Autodesk Fusion 360 part; units mm, degrees
note: some values were not read from the file. Chosen so that the rebuilt part matches the saved one: a side.
(part 2 of 2)
  spline S329 degree 2 poles (-148.7917, 5.9755) (-148.7208, 5.8468) (-148.7208, 5.7496) knots 0 0 0 1 1 1
  spline S330 degree 2 poles (-152.9965, 5.5659) (-152.9965, 5.6841) (-152.944, 5.9416) knots 0 0 0 1 1 1
  spline S331 degree 2 poles (-152.2034, 5.2611) (-151.8751, 5.2611) (-151.3288, 5.8134) knots 0 0 0 1 1 1
  spline S332 degree 2 poles (-160.0589, 6.9971) (-159.4128, 6.3957) (-159.4128, 5.9177) knots 0 0 0 1 1 1
  spline S333 degree 2 poles (-153.6965, 5.7036) (-153.3774, 6.0595) (-152.6498, 7.2204) knots 0 0 0 1 1 1
  spline S334 degree 2 poles (-164.6656, 7.3964) (-164.4713, 7.5592) (-164.2664, 7.5592) knots 0 0 0 1 1 1
  spline S335 degree 2 poles (-153.5323, 5.4568) (-154.0812, 4.8698) (-154.5041, 4.8698) knots 0 0 0 1 1 1
  spline S336 degree 2 poles (-158.3307, 4.1265) (-158.3964, 3.7982) (-158.3964, 3.5539) knots 0 0 0 1 1 1
  spline S337 degree 2 poles (-160.0563, 8.6465) (-160.3767, 8.6465) (-160.596, 8.4482) knots 0 0 0 1 1 1
  spline S338 degree 2 poles (-163.2684, 5.395) (-162.3806, 6.8002) (-162.3071, 7.8507) knots 0 0 0 1 1 1
  line L109 (-160.2953, 7.2151) -> (-160.0589, 6.9971)
  spline S339 degree 2 poles (-162.3071, 7.8507) (-161.8475, 7.7824) (-161.8475, 7.5434) knots 0 0 0 1 1 1
  spline S340 degree 2 poles (-158.7326, 3.1862) (-158.9506, 3.1862) (-158.9506, 3.4331) knots 0 0 0 1 1 1
  spline S341 degree 2 poles (-163.1528, 5.0667) (-163.7043, 4.313) (-164.248, 3.8783) knots 0 0 0 1 1 1
  line L110 (-152.944, 5.9416) -> (-152.8862, 6.2306)
  spline S342 degree 2 poles (-154.659, 9.3399) (-154.2625, 9.3399) (-153.9657, 9.5369) knots 0 0 0 1 1 1
  spline S343 degree 2 poles (-152.403, 6.0666) (-152.4791, 5.6967) (-152.4791, 5.5864) knots 0 0 0 1 1 1
  spline S344 degree 2 poles (-154.6564, 5.7916) (-154.6564, 5.3478) (-154.3307, 5.3478) knots 0 0 0 1 1 1
  spline S345 degree 2 poles (-158.0576, 5.5053) (-157.7923, 5.1954) (-157.4063, 5.1954) knots 0 0 0 1 1 1
  spline S346 degree 2 poles (-157.4063, 5.1954) (-156.944, 5.1954) (-156.6196, 5.5841) knots 0 0 0 1 1 1
  spline S347 degree 2 poles (-156.9571, 7.4305) (-157.3248, 7.4305) (-157.7556, 7.0155) knots 0 0 0 1 1 1
  spline S348 degree 2 poles (-154.5041, 4.8698) (-154.8114, 4.8698) (-155.0005, 5.1074) knots 0 0 0 1 1 1
  spline S349 degree 2 poles (-152.4791, 5.5864) (-152.4791, 5.2611) (-152.2034, 5.2611) knots 0 0 0 1 1 1
  line L111 (-153.9657, 9.5369) -> (-154.575, 6.3773)
  spline S350 degree 2 poles (-156.2953, 6.5296) (-156.2953, 6.9315) (-156.4791, 7.181) knots 0 0 0 1 1 1
  spline S351 degree 2 poles (-154.5881, 8.9696) (-154.6906, 8.9538) (-154.7667, 8.9538) knots 0 0 0 1 1 1
  spline S352 degree 2 poles (-150.4607, 5.1508) (-150.659, 5.4318) (-150.659, 5.8757) knots 0 0 0 1 1 1
  line L112 (-155.1108, 6.3379) -> (-154.5881, 8.9696)
  spline S353 degree 2 poles (-155.0005, 5.1074) (-155.1896, 5.3451) (-155.1896, 5.7286) knots 0 0 0 1 1 1
sketch "Sketch4" plane through (-20, 0, 0) normal (-1, 0, 0) x (0, -1, 0)
  spline S0 degree 2 poles (168.3547, 5.852) (168.3547, 5.4239) (168.5898, 5.1797) knots 0 0 0 1 1 1
  spline S1 degree 2 poles (171.6036, 3.5539) (171.6036, 3.399) (171.6719, 3.2729) knots 0 0 0 1 1 1
  spline S2 degree 2 poles (169.2398, 4.9354) (169.6075, 4.9354) (169.8781, 5.156) knots 0 0 0 1 1 1
  spline S3 degree 2 poles (158.6397, 5.7785) (158.6397, 6.6006) (159.1379, 7.2256) knots 0 0 0 1 1 1
  spline S4 degree 2 poles (171.1821, 7.9781) (171.0731, 8.0871) (171.0074, 8.3839) knots 0 0 0 1 1 1
  spline S5 degree 2 poles (158.8067, 5.118) (158.6397, 5.3661) (158.6397, 5.7785) knots 0 0 0 1 1 1
  line L0 (180.3679, 8.0608) -> (181.7546, 8.0608)
  spline S6 degree 2 poles (179.8741, 8.2426) (179.9949, 8.6482) (180.163, 8.7997) knots 0 0 0 1 1 1
  line L1 (179.7218, 7.722) -> (179.2779, 7.722)
  spline S7 degree 2 poles (177.6469, 8.4044) (177.8229, 8.4123) (178.1525, 8.5819) knots 0 0 0 1 1 1
  line L2 (177.6102, 8.4071) -> (177.6469, 8.4044)
  spline S8 degree 2 poles (173.71, 5.4712) (173.1978, 4.9354) (172.4939, 4.9354) knots 0 0 0 1 1 1
  spline S9 degree 2 poles (171.5905, 8.2552) (172.0763, 8.2552) (172.5255, 8.4338) knots 0 0 0 1 1 1
  spline S10 degree 2 poles (172.4939, 4.9354) (172.1131, 4.9354) (171.861, 5.0983) knots 0 0 0 1 1 1
  line L3 (172.5255, 8.4338) -> (172.3232, 7.42)
  line L4 (179.425, 8.0608) -> (179.8216, 8.0608)
  spline S11 degree 2 poles (175.425, 6.3773) (175.3436, 5.9518) (175.3436, 5.7916) knots 0 0 0 1 1 1
  spline S12 degree 2 poles (177.1532, 7.3523) (177.4946, 7.431) (177.5813, 7.431) knots 0 0 0 1 1 1
  spline S13 degree 2 poles (165.9805, 7.1258) (165.4158, 6.3694) (164.5071, 5.8599) knots 0 0 0 1 1 1
  spline S14 degree 2 poles (164.8853, 3.9348) (165.6548, 3.9348) (166.3561, 4.9512) knots 0 0 0 1 1 1
  spline S15 degree 2 poles (165.752, 3.8783) (165.2083, 3.4436) (164.817, 3.4436) knots 0 0 0 1 1 1
  line L5 (164.1368, 6.506) -> (164.3705, 6.0805)
  spline S16 degree 2 poles (163.3541, 7.1626) (163.3541, 7.6616) (163.9345, 7.9663) knots 0 0 0 1 1 1
  spline S17 degree 2 poles (163.0205, 4.6176) (162.8341, 4.7542) (162.8341, 4.9459) knots 0 0 0 1 1 1
  spline S18 degree 2 poles (164.5964, 5.4791) (164.5964, 5.0772) (164.2602, 4.7791) knots 0 0 0 1 1 1
  spline S19 degree 2 poles (163.2884, 4.9801) (163.2884, 4.7647) (163.601, 4.7647) knots 0 0 0 1 1 1
  spline S20 degree 2 poles (163.0901, 5.3609) (163.3462, 5.571) (163.9477, 5.8599) knots 0 0 0 1 1 1
  spline S21 degree 2 poles (163.601, 4.7647) (163.8321, 4.7647) (163.9765, 4.921) knots 0 0 0 1 1 1
  line L6 (163.9477, 5.8599) -> (163.7375, 6.1987)
  spline S22 degree 2 poles (164.0606, 5.6235) (163.2884, 5.2086) (163.2884, 4.9801) knots 0 0 0 1 1 1
  line L7 (163.4723, 7.2309) -> (163.6771, 7.0891)
  spline S23 degree 2 poles (164.5071, 5.8599) (164.5964, 5.6603) (164.5964, 5.4791) knots 0 0 0 1 1 1
  spline S24 degree 2 poles (162.8341, 4.9459) (162.8341, 5.1508) (163.0901, 5.3609) knots 0 0 0 1 1 1
  spline S25 degree 2 poles (163.7375, 6.1987) (163.3541, 6.8159) (163.3541, 7.1626) knots 0 0 0 1 1 1
  spline S26 degree 2 poles (164.2602, 4.7791) (163.924, 4.4811) (163.4723, 4.4811) knots 0 0 0 1 1 1
  spline S27 degree 2 poles (163.9345, 7.9663) (164.2917, 7.8297) (164.2917, 7.6222) knots 0 0 0 1 1 1
  spline S28 degree 2 poles (169.1847, 7.9584) (169.1847, 7.764) (169.2569, 7.6616) knots 0 0 0 1 1 1
  line L8 (171.861, 5.0983) -> (171.6693, 4.1265)
  spline S29 degree 2 poles (170.1486, 5.6734) (170.1486, 5.9912) (169.5524, 6.548) knots 0 0 0 1 1 1
  spline S30 degree 2 poles (168.7093, 7.764) (168.7093, 8.2683) (169.1033, 8.594) knots 0 0 0 1 1 1
  spline S31 degree 2 poles (169.035, 4.6281) (168.5859, 4.6281) (168.293, 4.8382) knots 0 0 0 1 1 1
  line L9 (169.5524, 6.548) -> (169.2635, 6.8159)
  spline S32 degree 2 poles (169.2635, 6.8159) (168.7093, 7.3307) (168.7093, 7.764) knots 0 0 0 1 1 1
  spline S33 degree 2 poles (166.3193, 6.7608) (166.5951, 6.007) (166.7316, 5.395) knots 0 0 0 1 1 1
  spline S34 degree 2 poles (171.0074, 8.3839) (171.1991, 8.2552) (171.5905, 8.2552) knots 0 0 0 1 1 1
  line L10 (165.7704, 7.2545) -> (165.9805, 7.1258)
  spline S35 degree 2 poles (170.687, 8.2053) (170.4585, 8.6465) (169.9437, 8.6465) knots 0 0 0 1 1 1
  spline S36 degree 2 poles (171.5196, 7.8691) (171.2911, 7.8691) (171.1821, 7.9781) knots 0 0 0 1 1 1
  spline S37 degree 2 poles (171.903, 7.9164) (171.6745, 7.8691) (171.5196, 7.8691) knots 0 0 0 1 1 1
  spline S38 degree 2 poles (169.8781, 5.156) (170.1486, 5.3767) (170.1486, 5.6734) knots 0 0 0 1 1 1
  spline S39 degree 2 poles (165.7336, 7.5592) (165.9096, 7.5592) (166.0264, 7.4003) knots 0 0 0 1 1 1
  spline S40 degree 2 poles (168.0002, 5.3688) (168.0002, 5.5868) (168.3547, 5.852) knots 0 0 0 1 1 1
  spline S41 degree 2 poles (171.6719, 3.2729) (171.4066, 3.1862) (171.2674, 3.1862) knots 0 0 0 1 1 1
  spline S42 degree 2 poles (168.293, 4.8382) (168.0002, 5.0484) (168.0002, 5.3688) knots 0 0 0 1 1 1
  spline S43 degree 2 poles (171.0494, 3.4331) (171.0494, 3.6248) (171.1361, 4.0608) knots 0 0 0 1 1 1
  spline S44 degree 2 poles (169.1033, 8.594) (169.4972, 8.9197) (170.1066, 8.9197) knots 0 0 0 1 1 1
  spline S45 degree 2 poles (170.1066, 8.9197) (170.4296, 8.9197) (170.6292, 8.8212) knots 0 0 0 1 1 1
  spline S46 degree 2 poles (170.1459, 4.9945) (169.7047, 4.6281) (169.035, 4.6281) knots 0 0 0 1 1 1
  spline S47 degree 2 poles (156.3941, 4.8382) (155.5353, 4.8382) (155.5353, 5.4082) knots 0 0 0 1 1 1
  spline S48 degree 2 poles (162.5662, 5.6432) (161.9411, 5.0641) (161.492, 5.0641) knots 0 0 0 1 1 1
  line L11 (156.4113, 7.2046) -> (156.9544, 7.2046)
  line L12 (156.6725, 8.4994) -> (156.4113, 7.2046)
  spline S49 degree 2 poles (162.5045, 6.0241) (162.9969, 6.4981) (163.4723, 7.2309) knots 0 0 0 1 1 1
  line L13 (157.5197, 8.4994) -> (156.6725, 8.4994)
  spline S50 degree 2 poles (156.8065, 5.2585) (157.4788, 5.2585) (157.991, 5.4975) knots 0 0 0 1 1 1
  spline S51 degree 2 poles (157.0245, 4.8973) (156.6148, 4.8382) (156.3941, 4.8382) knots 0 0 0 1 1 1
  line L14 (155.7743, 7.2046) -> (155.861, 7.2046)
  spline S52 degree 2 poles (156.1289, 5.6078) (156.1289, 5.2585) (156.8065, 5.2585) knots 0 0 0 1 1 1
  spline S53 degree 2 poles (157.5997, 5.0116) (157.4342, 4.9564) (157.0245, 4.8973) knots 0 0 0 1 1 1
  spline S54 degree 2 poles (155.5012, 8.7306) (155.6798, 8.8225) (156.6016, 8.8225) knots 0 0 0 1 1 1
  line L15 (156.1184, 8.4994) -> (156.0422, 8.4994)
  line L16 (155.7953, 6.879) -> (155.7559, 6.879)
  spline S55 degree 2 poles (155.4788, 7.1258) (155.5721, 7.2046) (155.7743, 7.2046) knots 0 0 0 1 1 1
  spline S56 degree 2 poles (155.5353, 5.4082) (155.5353, 5.5605) (155.6194, 5.9939) knots 0 0 0 1 1 1
  spline S57 degree 2 poles (159.5174, 5.3714) (159.8935, 5.3714) (160.956, 7.0208) knots 0 0 0 1 1 1
  spline S58 degree 2 poles (159.4596, 7.0457) (159.1702, 6.5638) (159.1702, 5.9019) knots 0 0 0 1 1 1
  spline S59 degree 2 poles (170.5872, 5.9177) (170.5872, 5.3609) (170.1459, 4.9945) knots 0 0 0 1 1 1
  spline S60 degree 2 poles (169.2569, 7.6616) (169.3291, 7.5592) (169.7047, 7.2151) knots 0 0 0 1 1 1
  spline S61 degree 2 poles (166.0264, 7.4003) (166.1433, 7.2414) (166.3193, 6.7608) knots 0 0 0 1 1 1
  spline S62 degree 2 poles (168.5898, 5.1797) (168.8249, 4.9354) (169.2398, 4.9354) knots 0 0 0 1 1 1
  spline S63 degree 2 poles (165.9555, 6.3445) (165.6679, 7.0339) (165.3344, 7.3964) knots 0 0 0 1 1 1
  spline S64 degree 2 poles (169.404, 8.4482) (169.1847, 8.2499) (169.1847, 7.9584) knots 0 0 0 1 1 1
  spline S65 degree 2 poles (168.1525, 7.5434) (168.1525, 7.2913) (167.7389, 6.506) knots 0 0 0 1 1 1
  spline S66 degree 2 poles (170.6292, 8.8212) (170.8288, 8.7227) (170.8288, 8.5651) knots 0 0 0 1 1 1
  spline S67 degree 2 poles (166.3561, 4.9512) (166.2431, 5.6551) (165.9555, 6.3445) knots 0 0 0 1 1 1
  spline S68 degree 2 poles (165.1269, 6.594) (165.3817, 6.808) (165.7704, 7.2545) knots 0 0 0 1 1 1
  spline S69 degree 2 poles (167.7389, 6.506) (167.3252, 5.7207) (166.8472, 5.0667) knots 0 0 0 1 1 1
  line L17 (171.1361, 4.0608) -> (171.903, 7.9164)
  spline S70 degree 2 poles (160.2908, 7.8507) (160.6878, 7.8507) (161.1505, 7.6038) knots 0 0 0 1 1 1
  spline S71 degree 2 poles (159.1379, 7.2256) (159.6361, 7.8507) (160.2908, 7.8507) knots 0 0 0 1 1 1
  spline S72 degree 2 poles (159.1702, 5.9019) (159.1702, 5.3714) (159.5174, 5.3714) knots 0 0 0 1 1 1
  spline S73 degree 2 poles (161.8098, 7.8455) (161.6601, 7.617) (161.5813, 7.2204) knots 0 0 0 1 1 1
  spline S74 degree 2 poles (160.956, 7.0208) (160.9692, 7.0418) (161.0639, 7.1679) knots 0 0 0 1 1 1
  spline S75 degree 2 poles (160.1109, 5.357) (159.6178, 4.8698) (159.2524, 4.8698) knots 0 0 0 1 1 1
  spline S76 degree 2 poles (159.2524, 4.8698) (158.9736, 4.8698) (158.8067, 5.118) knots 0 0 0 1 1 1
  spline S77 degree 2 poles (161.7073, 7.8481) (161.7389, 7.8481) (161.8098, 7.8455) knots 0 0 0 1 1 1
  spline S78 degree 2 poles (161.0639, 7.1679) (160.5115, 7.5277) (160.146, 7.5277) knots 0 0 0 1 1 1
  spline S79 degree 2 poles (161.1505, 7.6038) (161.2188, 7.8481) (161.7073, 7.8481) knots 0 0 0 1 1 1
  line L18 (161.5813, 7.2204) -> (161.5366, 6.9971)
  spline S80 degree 2 poles (160.9247, 6.0096) (160.9247, 6.2066) (160.9404, 6.5401) knots 0 0 0 1 1 1
  spline S81 degree 2 poles (161.7284, 5.55) (162.012, 5.55) (162.5045, 6.0241) knots 0 0 0 1 1 1
  spline S82 degree 2 poles (161.492, 5.0641) (160.9247, 5.0641) (160.9247, 6.0096) knots 0 0 0 1 1 1
  spline S83 degree 2 poles (161.5366, 6.9971) (161.4605, 6.6242) (161.4605, 6.1252) knots 0 0 0 1 1 1
  spline S84 degree 2 poles (160.146, 7.5277) (159.7489, 7.5277) (159.4596, 7.0457) knots 0 0 0 1 1 1
  spline S85 degree 2 poles (161.4605, 6.1252) (161.4605, 5.55) (161.7284, 5.55) knots 0 0 0 1 1 1
  spline S86 degree 2 poles (160.9404, 6.5401) (160.6039, 5.8442) (160.1109, 5.357) knots 0 0 0 1 1 1
  spline S87 degree 2 poles (164.3705, 6.0805) (164.8721, 6.3799) (165.1269, 6.594) knots 0 0 0 1 1 1
  line L19 (156.3479, 6.879) -> (156.2133, 6.204)
  spline S88 degree 2 poles (182.3114, 8.1557) (182.2458, 7.8866) (182.1368, 7.8043) knots 0 0 0 1 1 1
  spline S89 degree 2 poles (157.3843, 8.8225) (158.1249, 8.8225) (158.5872, 8.9696) knots 0 0 0 1 1 1
  spline S90 degree 2 poles (177.5813, 7.431) (177.7756, 7.431) (177.7756, 7.1581) knots 0 0 0 1 1 1
  spline S91 degree 2 poles (157.5447, 6.9472) (157.4056, 6.879) (156.8912, 6.879) knots 0 0 0 1 1 1
  line L20 (155.861, 7.2046) -> (156.1184, 8.4994)
  spline S92 degree 2 poles (156.9544, 7.2046) (157.5238, 7.2046) (157.8623, 7.3491) knots 0 0 0 1 1 1
  spline S93 degree 2 poles (156.2133, 6.204) (156.1289, 5.7837) (156.1289, 5.6078) knots 0 0 0 1 1 1
  spline S94 degree 2 poles (177.7756, 7.1581) (177.7756, 6.9561) (177.6995, 6.5782) knots 0 0 0 1 1 1
  spline S95 degree 2 poles (179.9477, 7.0847) (179.3541, 6.0442) (178.7474, 5.457) knots 0 0 0 1 1 1
  spline S96 degree 2 poles (178.6686, 8.9275) (178.553, 8.5651) (178.2589, 8.3208) knots 0 0 0 1 1 1
  line L21 (156.6016, 8.8225) -> (157.3843, 8.8225)
  line L22 (179.7297, 7.2132) -> (179.9477, 7.0847)
  spline S97 degree 2 poles (178.8341, 7.6432) (178.9864, 7.9199) (179.0862, 7.9904) knots 0 0 0 1 1 1
  spline S98 degree 2 poles (156.0422, 8.4994) (155.5563, 8.4994) (155.1414, 8.1895) knots 0 0 0 1 1 1
  spline S99 degree 2 poles (177.6548, 7.9479) (177.5498, 7.9479) (177.5498, 8.0765) knots 0 0 0 1 1 1
  line L23 (156.8912, 6.879) -> (156.3479, 6.879)
  spline S100 degree 2 poles (177.5498, 8.0765) (177.5498, 8.2601) (177.6102, 8.4071) knots 0 0 0 1 1 1
  spline S101 degree 2 poles (180.7934, 8.9459) (180.5885, 8.6825) (180.3679, 8.0608) knots 0 0 0 1 1 1
  line L24 (179.8216, 8.0608) -> (179.8741, 8.2426)
  spline S102 degree 2 poles (181.7546, 8.0608) (182.1197, 8.0608) (182.3114, 8.1557) knots 0 0 0 1 1 1
  spline S103 degree 2 poles (178.1525, 8.5819) (178.4821, 8.7514) (178.6686, 8.9275) knots 0 0 0 1 1 1
  spline S104 degree 2 poles (180.2549, 7.722) (180.2287, 7.6354) (180.2155, 7.5933) knots 0 0 0 1 1 1
  spline S105 degree 2 poles (180.163, 8.7997) (180.3311, 8.9512) (180.6673, 8.9512) knots 0 0 0 1 1 1
  spline S106 degree 2 poles (158.5872, 8.9696) (158.38, 8.6413) (158.2187, 8.5704) knots 0 0 0 1 1 1
  line L25 (177.3502, 7.2204) -> (177.5603, 7.0759)
  spline S107 degree 2 poles (155.7559, 6.879) (155.4907, 6.879) (155.2412, 6.7634) knots 0 0 0 1 1 1
  spline S108 degree 2 poles (179.0862, 7.9904) (179.186, 8.0608) (179.425, 8.0608) knots 0 0 0 1 1 1
  spline S109 degree 2 poles (158.2187, 8.5704) (158.0574, 8.4994) (157.5197, 8.4994) knots 0 0 0 1 1 1
  line L26 (181.731, 7.722) -> (180.2549, 7.722)
  spline S110 degree 2 poles (157.8623, 7.3491) (157.6838, 7.0155) (157.5447, 6.9472) knots 0 0 0 1 1 1
  spline S111 degree 2 poles (177.5603, 7.0759) (177.0166, 6.0438) (176.4677, 5.4568) knots 0 0 0 1 1 1
  spline S112 degree 2 poles (155.1414, 8.1895) (155.2727, 8.6097) (155.5012, 8.7306) knots 0 0 0 1 1 1
  spline S113 degree 2 poles (157.991, 5.4975) (157.8728, 5.1035) (157.5997, 5.0116) knots 0 0 0 1 1 1
  spline S114 degree 2 poles (179.341, 5.8757) (179.341, 6.3694) (179.601, 7.2808) knots 0 0 0 1 1 1
  line L27 (155.6194, 5.9939) -> (155.7953, 6.879)
  spline S115 degree 2 poles (177.1138, 6.2306) (177.2425, 6.8558) (177.2425, 7.108) knots 0 0 0 1 1 1
  spline S116 degree 2 poles (178.6712, 5.8134) (179.2175, 6.3657) (179.7297, 7.2132) knots 0 0 0 1 1 1
  spline S117 degree 2 poles (155.2412, 6.7634) (155.3856, 7.047) (155.4788, 7.1258) knots 0 0 0 1 1 1
  spline S118 degree 2 poles (180.2155, 7.5933) (179.8978, 6.5113) (179.8978, 5.9597) knots 0 0 0 1 1 1
  spline S119 degree 2 poles (179.2779, 7.722) (178.9995, 7.722) (178.8341, 7.6432) knots 0 0 0 1 1 1
  spline S120 degree 2 poles (178.2589, 8.3208) (177.8124, 7.9479) (177.6548, 7.9479) knots 0 0 0 1 1 1
  line L28 (172.2444, 7.0155) -> (171.9424, 5.5053)
  spline S121 degree 2 poles (182.1368, 7.8043) (182.0278, 7.722) (181.731, 7.722) knots 0 0 0 1 1 1
  spline S122 degree 2 poles (173.2477, 7.8507) (173.6653, 7.8507) (173.9437, 7.5342) knots 0 0 0 1 1 1
  line L29 (174.6292, 9.4581) -> (174.6292, 9.5185)
  spline S123 degree 2 poles (173.9437, 7.5342) (174.2221, 7.2178) (174.2221, 6.745) knots 0 0 0 1 1 1
  spline S124 degree 2 poles (174.2221, 6.745) (174.2221, 6.007) (173.71, 5.4712) knots 0 0 0 1 1 1
  spline S125 degree 2 poles (175.6693, 5.3478) (175.9844, 5.3478) (176.3035, 5.7036) knots 0 0 0 1 1 1
  spline S126 degree 2 poles (175.2333, 8.9538) (174.6292, 8.9538) (174.6292, 9.4581) knots 0 0 0 1 1 1
  spline S127 degree 2 poles (174.6292, 9.5185) (174.9444, 9.3399) (175.341, 9.3399) knots 0 0 0 1 1 1
  spline S128 degree 2 poles (180.6673, 8.9512) (180.7067, 8.9512) (180.7934, 8.9459) knots 0 0 0 1 1 1
  line L30 (179.601, 7.2808) -> (179.7218, 7.722)
  spline S129 degree 2 poles (177.2425, 7.108) (177.2425, 7.2577) (177.1532, 7.3523) knots 0 0 0 1 1 1
  spline S130 degree 2 poles (174.8104, 5.7286) (174.8104, 5.944) (174.8892, 6.3379) knots 0 0 0 1 1 1
  spline S131 degree 2 poles (173.3804, 5.5841) (173.7047, 5.9728) (173.7047, 6.5296) knots 0 0 0 1 1 1
  spline S132 degree 2 poles (172.3232, 7.42) (172.7697, 7.8507) (173.2477, 7.8507) knots 0 0 0 1 1 1
  spline S133 degree 2 poles (173.5209, 7.181) (173.337, 7.4305) (173.0429, 7.4305) knots 0 0 0 1 1 1
  spline S134 degree 2 poles (163.9765, 4.921) (164.121, 5.0772) (164.121, 5.3241) knots 0 0 0 1 1 1
  spline S135 degree 2 poles (164.2917, 7.6222) (164.2917, 7.3281) (163.8373, 7.0575) knots 0 0 0 1 1 1
  spline S136 degree 2 poles (163.6771, 7.0891) (163.1913, 6.2224) (162.5662, 5.6432) knots 0 0 0 1 1 1
  spline S137 degree 2 poles (164.817, 3.4436) (164.4651, 3.4436) (164.4651, 3.7404) knots 0 0 0 1 1 1
  line L31 (163.8373, 7.0575) -> (164.1368, 6.506)
  spline S138 degree 2 poles (164.5281, 4.0241) (164.6725, 3.9348) (164.8853, 3.9348) knots 0 0 0 1 1 1
  spline S139 degree 2 poles (164.121, 5.3241) (164.121, 5.4712) (164.0606, 5.6235) knots 0 0 0 1 1 1
  spline S140 degree 2 poles (163.4723, 4.4811) (163.207, 4.4811) (163.0205, 4.6176) knots 0 0 0 1 1 1
  spline S141 degree 2 poles (164.4651, 3.7404) (164.4651, 3.8612) (164.5281, 4.0241) knots 0 0 0 1 1 1
  spline S142 degree 2 poles (180.0527, 4.8698) (179.7375, 4.8698) (179.5393, 5.1508) knots 0 0 0 1 1 1
  spline S143 degree 2 poles (178.7474, 5.457) (178.1407, 4.8698) (177.6574, 4.8698) knots 0 0 0 1 1 1
  spline S144 degree 2 poles (177.1834, 5.0615) (177.0035, 5.2533) (177.0035, 5.5659) knots 0 0 0 1 1 1
  spline S145 degree 2 poles (181.2792, 5.7496) (181.2792, 5.4922) (180.8446, 5.181) knots 0 0 0 1 1 1
  spline S146 degree 2 poles (177.6574, 4.8698) (177.3633, 4.8698) (177.1834, 5.0615) knots 0 0 0 1 1 1
  spline S147 degree 2 poles (180.3364, 5.3504) (180.5622, 5.3504) (180.8288, 5.5421) knots 0 0 0 1 1 1
  spline S148 degree 2 poles (170.8288, 8.5651) (170.8288, 8.4101) (170.687, 8.2053) knots 0 0 0 1 1 1
  spline S149 degree 2 poles (180.8288, 5.5421) (181.0954, 5.7338) (181.2083, 5.9755) knots 0 0 0 1 1 1
  line L32 (177.6995, 6.5782) -> (177.597, 6.0666)
  spline S150 degree 2 poles (180.8446, 5.181) (180.4099, 4.8698) (180.0527, 4.8698) knots 0 0 0 1 1 1
  spline S151 degree 2 poles (179.8978, 5.9597) (179.8978, 5.3504) (180.3364, 5.3504) knots 0 0 0 1 1 1
  spline S152 degree 2 poles (181.2083, 5.9755) (181.2792, 5.8468) (181.2792, 5.7496) knots 0 0 0 1 1 1
  spline S153 degree 2 poles (177.0035, 5.5659) (177.0035, 5.6841) (177.056, 5.9416) knots 0 0 0 1 1 1
  spline S154 degree 2 poles (177.7966, 5.2611) (178.1249, 5.2611) (178.6712, 5.8134) knots 0 0 0 1 1 1
  spline S155 degree 2 poles (169.9411, 6.9971) (170.5872, 6.3957) (170.5872, 5.9177) knots 0 0 0 1 1 1
  spline S156 degree 2 poles (176.3035, 5.7036) (176.6226, 6.0595) (177.3502, 7.2204) knots 0 0 0 1 1 1
  spline S157 degree 2 poles (165.3344, 7.3964) (165.5287, 7.5592) (165.7336, 7.5592) knots 0 0 0 1 1 1
  spline S158 degree 2 poles (176.4677, 5.4568) (175.9188, 4.8698) (175.4959, 4.8698) knots 0 0 0 1 1 1
  spline S159 degree 2 poles (171.6693, 4.1265) (171.6036, 3.7982) (171.6036, 3.5539) knots 0 0 0 1 1 1
  spline S160 degree 2 poles (169.9437, 8.6465) (169.6233, 8.6465) (169.404, 8.4482) knots 0 0 0 1 1 1
  spline S161 degree 2 poles (166.7316, 5.395) (167.6194, 6.8002) (167.6929, 7.8507) knots 0 0 0 1 1 1
  line L33 (169.7047, 7.2151) -> (169.9411, 6.9971)
  spline S162 degree 2 poles (167.6929, 7.8507) (168.1525, 7.7824) (168.1525, 7.5434) knots 0 0 0 1 1 1
  spline S163 degree 2 poles (171.2674, 3.1862) (171.0494, 3.1862) (171.0494, 3.4331) knots 0 0 0 1 1 1
  spline S164 degree 2 poles (166.8472, 5.0667) (166.2957, 4.313) (165.752, 3.8783) knots 0 0 0 1 1 1
  line L34 (177.056, 5.9416) -> (177.1138, 6.2306)
  spline S165 degree 2 poles (175.341, 9.3399) (175.7375, 9.3399) (176.0343, 9.5369) knots 0 0 0 1 1 1
  spline S166 degree 2 poles (177.597, 6.0666) (177.5209, 5.6967) (177.5209, 5.5864) knots 0 0 0 1 1 1
  spline S167 degree 2 poles (175.3436, 5.7916) (175.3436, 5.3478) (175.6693, 5.3478) knots 0 0 0 1 1 1
  spline S168 degree 2 poles (171.9424, 5.5053) (172.2077, 5.1954) (172.5937, 5.1954) knots 0 0 0 1 1 1
  spline S169 degree 2 poles (172.5937, 5.1954) (173.056, 5.1954) (173.3804, 5.5841) knots 0 0 0 1 1 1
  spline S170 degree 2 poles (173.0429, 7.4305) (172.6752, 7.4305) (172.2444, 7.0155) knots 0 0 0 1 1 1
  spline S171 degree 2 poles (175.4959, 4.8698) (175.1886, 4.8698) (174.9995, 5.1074) knots 0 0 0 1 1 1
  spline S172 degree 2 poles (177.5209, 5.5864) (177.5209, 5.2611) (177.7966, 5.2611) knots 0 0 0 1 1 1
  line L35 (176.0343, 9.5369) -> (175.425, 6.3773)
  spline S173 degree 2 poles (173.7047, 6.5296) (173.7047, 6.9315) (173.5209, 7.181) knots 0 0 0 1 1 1
  spline S174 degree 2 poles (175.4119, 8.9696) (175.3094, 8.9538) (175.2333, 8.9538) knots 0 0 0 1 1 1
  spline S175 degree 2 poles (179.5393, 5.1508) (179.341, 5.4318) (179.341, 5.8757) knots 0 0 0 1 1 1
  line L36 (174.8892, 6.3379) -> (175.4119, 8.9696)
  spline S176 degree 2 poles (174.9995, 5.1074) (174.8104, 5.3451) (174.8104, 5.7286) knots 0 0 0 1 1 1
extrude "Extrude5" cut sketch "Sketch3" against normal blind 0.8 thin wall 1 on the left open curves L12 L6 L26 L24 L7
extrude "Extrude6" cut sketch "Sketch4" against normal blind 4 contours S0 S2 S28 S29 S30 S31 L9 S32 S35 S38 S40 S42 S44 S45 S46 S59 S60 S62 S64 S66 S148 S155 S160 L33 | S1 S4 S8 S9 S10 L3 L8 S34 S36 S37 S41 S43 L17 S122 S123 S124 S132 S159 S163 | S3 S5 S25 S48 S49 S70 S71 S73 S75 S76 S77 S79 L18 S80 S81 S82 S83 S85 S86 S136 | S13 L5 S16 S17 S18 S20 L6 L7 S23 S24 S25 S26 S27 S49 S63 S68 S87 S135 S136 L31 S140 | S13 S14 S15 S33 L10 S39 S61 S63 S65 S67 S68 S69 S137 S138 S141 S157 S161 S162 S164 | L0 S6 L1 L4 S88 S95 L22 S97 S101 L24 S102 S104 S105 S108 L26 S114 S116 S118 S119 S121 S128 L30 S142 S145 S147 S149 S150 S151 S152 S175 | S12 S90 S94 S95 L25 S111 S114 S115 S116 S129 S143 S144 S146 L32 S153 S154 S156 L34 S166 S172 | S11 S111 S115 L29 S125 S126 S127 S130 S156 S158 S165 S167 S171 L35 S174 L36 S176 | S7 L2 S96 S99 S100 S103 S120 | S47 L11 L12 L13 S50 S51 L14 S52 S53 S54 L15 L16 S55 S56 L19 S89 S91 L20 S92 S93 L21 S98 L23 S106 S107 S109 S110 S112 S113 L27 S117
extrude "Extrude7" cut sketch "Sketch3" against normal blind 4 thin wall 1 on the left open curves L38 L4 L13 L23 L15 L28 L30 L9 L18 L17 L29 L25 L27 L8 L10 L14 L22 L21 L20 L11 L19 L16 L5 L31 L32 L33 L34 L35 L36 L37
sketch "Sketch5" plane through (0, 0, 13) normal (0, 0, 1) x (-1, 0, 0)
  line L0 (16, -5.5) -> (20, -5.5)
  line L1 (20, -5.5) -> (20, -0.6491)
  line L2 (20, -0.6491) -> (16, -0.6491)
  line L3 (16, -0.6491) -> (16, 0.5)
  line L4 (16, 0.5) -> (20, 0.5)
  line L5 (20, 0.5) -> (20, 5.3509)
  line L6 (20, 5.3509) -> (16, 5.3509)
  line L7 (16, 5.3509) -> (16, 6.5)
  line L8 (16, 6.5) -> (20, 6.5)
  line L9 (20, 6.5) -> (20, 11.3509)
  line L10 (20, 11.3509) -> (16, 11.3509)
  line L11 (16, 11.3509) -> (16, 12.5)
  line L12 (16, 12.5) -> (20, 12.5)
  line L13 (20, 12.5) -> (20, 17.3509)
  line L14 (20, 17.3509) -> (16, 17.3509)
  line L15 (16, 17.3509) -> (16, 18.5)
  line L16 (16, 18.5) -> (20, 18.5)
  line L17 (20, 18.5) -> (20, 23.3509)
  line L18 (20, 23.3509) -> (16, 23.3509)
  line L19 (16, 23.3509) -> (16, 24.5)
  line L20 (16, 24.5) -> (20, 24.5)
  line L21 (20, 24.5) -> (20, 29.3509)
  line L22 (20, 29.3509) -> (16, 29.3509)
  line L23 (16, 29.3509) -> (16, 30.5)
  line L24 (16, 30.5) -> (20, 30.5)
  line L25 (20, 30.5) -> (20, 35.3509)
  line L26 (20, 35.3509) -> (16, 35.3509)
  line L27 (16, 35.3509) -> (16, 36.5)
  line L28 (16, 36.5) -> (20, 36.5)
  line L29 (20, 36.5) -> (20, 41.3509)
  line L30 (20, 41.3509) -> (16, 41.3509)
  line L31 (16, 41.3509) -> (16, 42.5)
  line L32 (16, 42.5) -> (20, 42.5)
  line L33 (20, 42.5) -> (20, 47.3509)
  line L34 (20, 47.3509) -> (16, 47.3509)
  line L35 (16, 47.3509) -> (16, 48.5)
  line L36 (16, 48.5) -> (20, 48.5)
  line L37 (20, 48.5) -> (20, 53.3509)
  line L38 (20, 53.3509) -> (16, 53.3509)
  line L39 (16, 53.3509) -> (16, 54.5)
  line L40 (16, 54.5) -> (20, 54.5)
  line L41 (20, 54.5) -> (20, 59.3509)
  line L42 (20, 59.3509) -> (16, 59.3509)
  line L43 (16, 59.3509) -> (16, 60.5)
  line L44 (16, 60.5) -> (20, 60.5)
  line L45 (20, 60.5) -> (20, 65.3509)
  line L46 (20, 65.3509) -> (16, 65.3509)
  line L47 (16, 65.3509) -> (16, 66.5)
  line L48 (16, 66.5) -> (20, 66.5)
  line L49 (20, 66.5) -> (20, 71.3509)
  line L50 (20, 71.3509) -> (16, 71.3509)
  line L51 (16, 71.3509) -> (16, 72.5)
  line L52 (16, 72.5) -> (20, 72.5)
  line L53 (20, 72.5) -> (20, 77.3509)
  line L54 (20, 77.3509) -> (16, 77.3509)
  line L55 (16, 77.3509) -> (16, 78.5)
  line L56 (16, 78.5) -> (20, 78.5)
  line L57 (20, 78.5) -> (20, 83.3509)
  line L58 (20, 83.3509) -> (16, 83.3509)
  line L59 (16, 83.3509) -> (16, 84.5)
  line L60 (16, 84.5) -> (20, 84.5)
  line L61 (20, 84.5) -> (20, 89.3509)
  line L62 (20, 89.3509) -> (16, 89.3509)
  line L63 (16, 89.3509) -> (16, 90.5)
  line L64 (16, 90.5) -> (20, 90.5)
  line L65 (20, 90.5) -> (20, 95.3509)
  line L66 (20, 95.3509) -> (16, 95.3509)
  line L67 (16, 95.3509) -> (16, 96.5)
  line L68 (16, 96.5) -> (20, 96.5)
  line L69 (20, 96.5) -> (20, 101.3509)
  line L70 (20, 101.3509) -> (16, 101.3509)
  line L71 (16, 101.3509) -> (16, 102.5)
  line L72 (16, 102.5) -> (20, 102.5)
  line L73 (20, 102.5) -> (20, 107.3509)
  line L74 (20, 107.3509) -> (16, 107.3509)
  line L75 (16, 107.3509) -> (16, 108.5)
  line L76 (16, 108.5) -> (20, 108.5)
  line L77 (20, 108.5) -> (20, 113.3509)
  line L78 (20, 113.3509) -> (16, 113.3509)
  line L79 (16, 113.3509) -> (16, 114.5)
  line L80 (16, 114.5) -> (20, 114.5)
  line L81 (20, 114.5) -> (20, 119.3509)
  line L82 (20, 119.3509) -> (16, 119.3509)
  line L83 (16, 119.3509) -> (16, 120.5)
  line L84 (16, 120.5) -> (20, 120.5)
  line L85 (20, 120.5) -> (20, 125.3509)
  line L86 (20, 125.3509) -> (16, 125.3509)
  line L87 (16, 125.3509) -> (16, 126.5)
  line L88 (16, 126.5) -> (20, 126.5)
  line L89 (20, 126.5) -> (20, 131.3509)
  line L90 (20, 131.3509) -> (16, 131.3509)
  line L91 (16, 131.3509) -> (16, 132.5)
  line L92 (16, 132.5) -> (20, 132.5)
  line L93 (20, 132.5) -> (20, 137.3509)
  line L94 (20, 137.3509) -> (16, 137.3509)
  line L95 (16, 137.3509) -> (16, 138.5)
  line L96 (16, 138.5) -> (20, 138.5)
  line L97 (20, 138.5) -> (20, 143.3509)
  line L98 (20, 143.3509) -> (16, 143.3509)
  line L99 (16, 143.3509) -> (16, 144.5)
  line L100 (16, 144.5) -> (20, 144.5)
  line L101 (20, 144.5) -> (20, 149.3509)
  line L102 (20, 149.3509) -> (16, 149.3509)
  line L103 (16, 149.3509) -> (16, 150.5)
  line L104 (16, 150.5) -> (20, 150.5)
  line L105 (20, 150.5) -> (20, 155.3509)
  line L106 (20, 155.3509) -> (16, 155.3509)
  line L107 (16, 155.3509) -> (16, 156.5)
  line L108 (16, 156.5) -> (20, 156.5)
  line L109 (20, 156.5) -> (20, 161.3509)
  line L110 (20, 161.3509) -> (19.2, 161.3509)
  line L111 (19.2, 161.3509) -> (19.2, 162.5)
  line L112 (19.2, 162.5) -> (20, 162.5)
  line L113 (20, 162.5) -> (20, 167.3509)
  line L114 (20, 167.3509) -> (19.2, 167.3509)
  line L115 (19.2, 167.3509) -> (19.2, 168.5)
  line L116 (19.2, 168.5) -> (20, 168.5)
  line L117 (20, 168.5) -> (20, 173.3509)
  line L118 (20, 173.3509) -> (19.2, 173.3509)
  line L119 (19.2, 173.3509) -> (19.2, 174.5)
  line L120 (19.2, 174.5) -> (20, 174.5)
  line L121 (20, 174.5) -> (20, 179.3509)
  line L122 (20, 179.3509) -> (19.2, 179.3509)
  line L123 (19.2, 179.3509) -> (19.2, 180.5)
  line L124 (19.2, 180.5) -> (20, 180.5)
  line L125 (20, 180.5) -> (20, 185.3509)
  line L126 (20, 185.3509) -> (19.2, 185.3509)
  line L127 (19.2, 185.3509) -> (19.2, 186.5)
  line L128 (19.2, 186.5) -> (20, 186.5)
  line L129 (20, 186.5) -> (20, 187.6438)
  arc A0 (20, 187.6438) -> (18.7178, 191.3509) centre (14, 187.6438) ccw
  line L130 (18.7178, 191.3509) -> (16, 191.3509)
  line L131 (16, 191.3509) -> (16, 192.5)
  line L132 (16, 192.5) -> (17.5238, 192.5)
  arc A1 (17.5238, 192.5) -> (14, 193.6438) centre (14, 187.6438) ccw
  line L133 (14, 193.6438) -> (-132.6875, 193.6438)
  line L134 (-132.6875, 193.6438) -> (-132.6875, 183.6438)
  line L135 (-132.6875, 183.6438) -> (10, 183.6438)
  line L136 (10, 183.6438) -> (10, -15)
  line L137 (10, -15) -> (-157.6875, -15)
  line L138 (-157.6875, -15) -> (-157.6875, 183.6438)
  line L139 (-157.6875, 183.6438) -> (-152.6875, 183.6438)
  line L140 (-152.6875, 183.6438) -> (-152.6875, 193.6438)
  line L141 (-152.6875, 193.6438) -> (-161.6875, 193.6438)
  arc A2 (-161.6875, 193.6438) -> (-167.6875, 187.6438) centre (-161.6875, 187.6438) ccw
  line L142 (-167.6875, 187.6438) -> (-167.6875, -19)
  arc A3 (-167.6875, -19) -> (-161.6875, -25) centre (-161.6875, -19) ccw
  line L143 (-161.6875, -25) -> (14, -25)
  arc A4 (14, -25) -> (20, -19) centre (14, -19) ccw
  line L144 (20, -19) -> (20, -12.6491)
  line L145 (20, -12.6491) -> (16, -12.6491)
  line L146 (16, -12.6491) -> (16, -11.5)
  line L147 (16, -11.5) -> (20, -11.5)
  line L148 (20, -11.5) -> (20, -6.6491)
  line L149 (20, -6.6491) -> (16, -6.6491)
  line L150 (16, -6.6491) -> (16, -5.5)
  circle A5 centre (14, -19) radius 2.2
  circle A6 centre (-161.6875, -19) radius 2.2
  circle A7 centre (14, 187.6438) radius 2.2
  circle A8 centre (-161.6875, 187.6438) radius 2.2
  dimension "d30" = 4.4
  dimension "d31" = 6
  dimension "d32" = 6
  dimension "d33" = 4.4
  dimension "d34" = 4.4
  dimension "d35" = 4.4
  dimension "d36" = 6
  dimension "d37" = 6
  dimension "d38" = 6
  dimension "d39" = 6
  dimension "d40" = 6
  dimension "d41" = 6
  measures "d30" diameter of A5
  measures "d31" distance of L144 A4.centre
  measures "d32" distance of L143 A4.centre
  measures "d33" diameter of A6
  measures "d34" diameter of A7
  measures "d35" diameter of A8
  measures "d36" distance of L141 A2.centre
  measures "d37" distance of L142 A2.centre
  measures "d38" distance of L133 A0.centre
  measures "d39" distance of L125 A0.centre
  measures "d40" distance of L143 A3.centre
  measures "d41" distance of L142 A3.centre
extrude "Extrude8" cut sketch "Sketch5" against normal blind 6 contours A5 | A6 | A7 | A8
